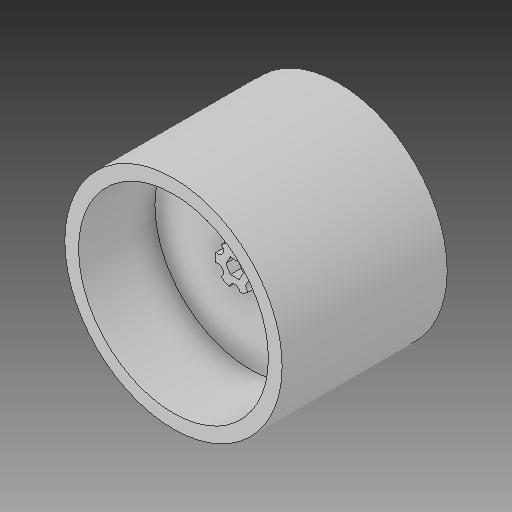
# Autodesk Inventor part: Wheel_Rim
Saved by Autodesk Inventor 2019 (Build 230136000, 136)
## iProperties
Created: 2019-03-02
Part Number: Wheel_Rim
Material: Generic
Document SubType Name: Modeling
Designer: alarr
Density: 1 g/cm^3
Appearance: Default
Author: alarr
Autodesk Inventor part; units mm, degrees
ref_plane "YZ Plane" through (0, 0, 0) normal (1, 0, 0) x (0, 1, 0)
ref_plane "XZ Plane" through (0, 0, 0) normal (0, 1, 0) x (-1, 0, 0)
ref_plane "XY Plane" through (0, 0, 0) normal (0, 0, 1) x (1, 0, 0)
sketch "Sketch1" plane through (0, 0, 0) normal (0, 0, 1) x (1, 0, 0)
  circle A0 centre (0, 0) radius 50.165
  dimension "d0" = 100.33
  constraints: 1 centre point, 1 coincident
  measures "d0" diameter of A0
extrude "Extrusion1" add sketch "Sketch1" along normal mid plane 76.2
sketch "Sketch2" plane through (0, 0, 38.1) normal (0, 0, 1) x (1, 0, 0)
  circle A0 centre (0, 0) radius 43.815
  dimension "d3" = 87.63
  constraints: 1 centre point, 1 coincident
  measures "d3" diameter of A0
extrude "Extrusion2" cut sketch "Sketch2" against normal through all
sketch "Sketch3" plane through (0, 0, 0) normal (0, 0, 1) x (1, 0, 0)
  circle A0 centre (0, 0) radius 43.815 projected
  circle A1 centre (0, 0) radius 43.815
  constraints: 1 centre point, 1 coincident, 1 concentric
extrude "Extrusion3" add sketch "Sketch3" along normal mid plane 5.715
sketch "Sketch4" plane through (0, 0, 2.8575) normal (0, 0, 1) x (1, 0, 0)
  arc A0 (-8.648, 2.06) -> (-8.648, -2.06) centre (0, 0) ccw
  arc A1 (-2.54, 8.5194) -> (2.54, 8.5194) centre (0, 8.89) ccw
  line L0 (0, 0) -> (0, 8.89) construction
  line L1 (-2.54, 8.5194) -> (2.54, 8.5194) construction
  arc A2 (-8.648, 2.06) -> (-6.108, 6.4594) centre (-7.699, 4.445) ccw
  arc A3 (-6.108, -6.4594) -> (-8.648, -2.06) centre (-7.699, -4.445) ccw
  arc A4 (2.54, -8.5194) -> (-2.54, -8.5194) centre (0, -8.89) ccw
  arc A5 (8.648, -2.06) -> (6.108, -6.4594) centre (7.699, -4.445) ccw
  arc A6 (6.108, 6.4594) -> (8.648, 2.06) centre (7.699, 4.445) ccw
  arc A7 (-6.108, 6.4594) -> (-8.648, 2.06) centre (0, 0) ccw construction
  arc A8 (8.648, 2.06) -> (6.108, 6.4594) centre (0, 0) ccw construction
  arc A9 (6.108, 6.4594) -> (-6.108, 6.4594) centre (0, 0) ccw
  arc A10 (8.648, -2.06) -> (8.648, 2.06) centre (0, 0) ccw
  arc A11 (6.108, -6.4594) -> (8.648, -2.06) centre (0, 0) ccw construction
  arc A12 (2.54, -8.5194) -> (6.108, -6.4594) centre (0, 0) ccw
  arc A13 (-2.54, -8.5194) -> (2.54, -8.5194) centre (0, 0) ccw construction
  arc A14 (-6.108, -6.4594) -> (-2.54, -8.5194) centre (0, 0) ccw
  arc A15 (-8.648, -2.06) -> (-6.108, -6.4594) centre (0, 0) ccw construction
  dimension "d8" = 17.78
  dimension "d10" = 5.08
  dimension "d13" = 360
  constraints: 41 point on circle, 16 centre point, 4 end point, 1 coincident, 1 horizontal, 1 vertical, 25 other
  measures "d8" diameter of A0
  measures "d10" distance of L1.end L1.start
extrude "Extrusion4" add sketch "Sketch4" along normal blind 6.985 contours A2 A9 A1 A6 A10 A5 A12 A4 A14 A3 A0
sketch "Sketch5" plane through (0, 0, 9.8425) normal (0, 0, 1) x (1, 0, 0)
  line L0 (-2.0164, 3.4925) -> (2.0164, 3.4925)
  line L1 (2.0164, 3.4925) -> (4.0328, 0)
  line L2 (4.0328, 0) -> (2.0164, -3.4925)
  line L3 (2.0164, -3.4925) -> (-2.0164, -3.4925)
  line L4 (-2.0164, -3.4925) -> (-4.0328, 0)
  line L5 (-4.0328, 0) -> (-2.0164, 3.4925)
  point P0 (0, 0)
  point P1 (0, 0)
  dimension "d17" = 6.985
  constraints: 12 end point, 1 coincident, 1 horizontal, 13 other
  measures "d17" distance between parallel lines of L3 L0
extrude "Extrusion5" cut sketch "Sketch5" against normal through all
body "Solid1"
